Autodesk Fusion 360 part; units mm, degrees
(part 2 of 2)
sketch "oled" plane through (0, 0, 8) normal (0, 0, 1) x (-1, 0, 0)
  line L0 (-139.875, 29.334375) -> (-144.098992, 29.334375)
  line L1 (-144.644364, 25.834375) -> (-139.875, 25.834375)
  line L2 (-139.875, 25.834375) -> (-139.875, 23.834375)
  line L3 (-139.875, 23.834375) -> (-144.91061, 23.834375)
  line L4 (-145.297865, 20.334375) -> (-139.875, 20.334375)
  line L5 (-139.875, 20.334375) -> (-139.875, 18.334375)
  line L6 (-139.875, 18.334375) -> (-145.474496, 18.334375)
  line L7 (-145.705944, 14.834375) -> (-139.875, 14.834375)
  line L8 (-139.875, 14.834375) -> (-139.875, 12.834375)
  line L9 (-139.875, 12.834375) -> (-145.794002, 12.834375)
  line L10 (-145.871001, 9.334375) -> (-139.875, 9.334375)
  line L11 (-139.875, 9.334375) -> (-139.875, 7.334375)
  line L12 (-139.875, 7.334375) -> (-145.871001, 7.334375)
  line L13 (-145.794002, 3.834375) -> (-139.875, 3.834375)
  line L14 (-139.875, 3.834375) -> (-139.875, 1.834375)
  line L15 (-139.875, 1.834375) -> (-145.705944, 1.834375)
  line L16 (-145.474496, -1.665625) -> (-139.875, -1.665625)
  line L17 (-139.875, -1.665625) -> (-139.875, -3.665625)
  line L18 (-139.875, -3.665625) -> (-145.297865, -3.665625)
  line L19 (-144.91061, -7.165625) -> (-139.875, -7.165625)
  line L20 (-139.875, -7.165625) -> (-139.875, -9.165625)
  line L21 (-139.875, -9.165625) -> (-144.644364, -9.165625)
  line L22 (-144.098992, -12.665625) -> (-139.875, -12.665625)
  line L23 (-139.875, -12.665625) -> (-139.875, -14.665625)
  line L24 (-139.875, -14.665625) -> (-143.741524, -14.665625)
  line L25 (-143.034704, -18.165625) -> (-139.875, -18.165625)
  line L26 (-139.875, -18.165625) -> (-139.875, -20.165625)
  line L27 (-139.875, -20.165625) -> (-142.583799, -20.165625)
  line L28 (9.233799, -20.165625) -> (6.525, -20.165625)
  line L29 (6.525, -20.165625) -> (6.525, -18.165625)
  line L30 (6.525, -18.165625) -> (9.684704, -18.165625)
  line L31 (10.391524, -14.665625) -> (6.525, -14.665625)
  line L32 (6.525, -14.665625) -> (6.525, -12.665625)
  line L33 (6.525, -12.665625) -> (10.748992, -12.665625)
  line L34 (11.294364, -9.165625) -> (6.525, -9.165625)
  line L35 (6.525, -9.165625) -> (6.525, -7.165625)
  line L36 (6.525, -7.165625) -> (11.56061, -7.165625)
  line L37 (11.947865, -3.665625) -> (6.525, -3.665625)
  line L38 (6.525, -3.665625) -> (6.525, -1.665625)
  line L39 (6.525, -1.665625) -> (12.124496, -1.665625)
  line L40 (12.355944, 1.834375) -> (6.525, 1.834375)
  line L41 (6.525, 1.834375) -> (6.525, 3.834375)
  line L42 (6.525, 3.834375) -> (12.444002, 3.834375)
  line L43 (12.521001, 7.334375) -> (6.525, 7.334375)
  line L44 (6.525, 7.334375) -> (6.525, 9.334375)
  line L45 (6.525, 9.334375) -> (12.521001, 9.334375)
  line L46 (12.444002, 12.834375) -> (6.525, 12.834375)
  line L47 (6.525, 12.834375) -> (6.525, 14.834375)
  line L48 (6.525, 14.834375) -> (12.355944, 14.834375)
  line L49 (12.124496, 18.334375) -> (6.525, 18.334375)
  line L50 (6.525, 18.334375) -> (6.525, 20.334375)
  line L51 (6.525, 20.334375) -> (11.947865, 20.334375)
  line L52 (11.56061, 23.834375) -> (6.525, 23.834375)
  line L53 (6.525, 23.834375) -> (6.525, 25.834375)
  line L54 (6.525, 25.834375) -> (11.294364, 25.834375)
  line L55 (10.748992, 29.334375) -> (6.525, 29.334375)
  line L56 (6.525, 29.334375) -> (6.525, 31.334375)
  line L57 (6.525, 31.334375) -> (10.391524, 31.334375)
  line L58 (9.684704, 34.834375) -> (6.525, 34.834375)
  line L59 (6.525, 34.834375) -> (6.525, 36.834375)
  line L60 (6.525, 36.834375) -> (9.233799, 36.834375)
  line L61 (0.525, 41.625) -> (0.525, 19.525)
  arc A0 (-0.475, 18.525) -> (0.525, 19.525) centre (-0.475, 19.525) ccw
  line L62 (-0.475, 18.525) -> (-9, 18.525)
  line L63 (-9, 18.525) -> (-9, 0.475)
  arc A1 (-10, -0.525) -> (-9, 0.475) centre (-10, 0.475) ccw
  line L64 (-10, -0.525) -> (-47.15, -0.525)
  arc A2 (-48.15, 0.475) -> (-47.15, -0.525) centre (-47.15, 0.475) ccw
  line L65 (-48.15, 0.475) -> (-48.15, 18.525)
  line L66 (-48.15, 18.525) -> (-66.15, 18.525)
  line L67 (-66.15, 18.525) -> (-66.15, 0.475)
  arc A3 (-67.15, -0.525) -> (-66.15, 0.475) centre (-67.15, 0.475) ccw
  line L68 (-67.15, -0.525) -> (-123.35, -0.525)
  arc A4 (-124.35, 0.475) -> (-123.35, -0.525) centre (-123.35, 0.475) ccw
  line L69 (-124.35, 0.475) -> (-124.35, 18.525)
  line L70 (-124.35, 18.525) -> (-132.875, 18.525)
  arc A5 (-133.875, 19.525) -> (-132.875, 18.525) centre (-132.875, 19.525) ccw
  line L71 (-133.875, 19.525) -> (-133.875, 41.625)
  line L72 (-142.583799, 36.834375) -> (-139.875, 36.834375)
  line L73 (-139.875, 36.834375) -> (-139.875, 34.834375)
  line L74 (-139.875, 34.834375) -> (-143.034704, 34.834375)
  line L75 (-143.741524, 31.334375) -> (-139.875, 31.334375)
  line L76 (-139.875, 31.334375) -> (-139.875, 29.334375)
  circle A6 centre (-123.825, -13.096875) radius 10
  line L77 (-15.876065, -17.914896) -> (-3.386093, -17.890586)
  arc A7 (-3.381227, -20.390581) -> (-3.386093, -17.890586) centre (-3.38366, -19.140584) ccw
  line L78 (-3.381227, -20.390581) -> (-15.871199, -20.414891)
  arc A8 (-15.876065, -17.914896) -> (-15.871199, -20.414891) centre (-15.873632, -19.164893) ccw
  line L79 (-15.877503, -5.914899) -> (-3.387616, -5.876226)
  arc A9 (-3.379875, -8.376214) -> (-3.387616, -5.876226) centre (-3.383745, -7.12622) ccw
  line L80 (-3.379875, -8.376214) -> (-15.869762, -8.414887)
  arc A10 (-15.877503, -5.914899) -> (-15.869762, -8.414887) centre (-15.873632, -7.164893) ccw
  line L81 (-18.024549, -13.914894) -> (-1.172265, -13.895698)
  arc A11 (-1.169417, -16.395696) -> (-1.172265, -13.895698) centre (-1.170841, -15.145697) ccw
  line L82 (-1.169417, -16.395696) -> (-18.021701, -16.414893)
  arc A12 (-18.024549, -13.914894) -> (-18.021701, -16.414893) centre (-18.023125, -15.164893) ccw
  line L83 (-18.024544, -9.914894) -> (-1.172264, -9.895769)
  arc A13 (-1.169426, -12.395767) -> (-1.172264, -9.895768) centre (-1.170845, -11.145768) ccw
  line L84 (-1.169426, -12.395767) -> (-18.021707, -12.414893)
  arc A14 (-18.024544, -9.914894) -> (-18.021707, -12.414893) centre (-18.023125, -11.164893) ccw
  line L85 (-106.15, -6.096875) -> (-75.15, -6.096875)
  line L86 (-75.15, -20.096875) -> (-75.15, -6.096875)
  line L87 (-106.15, -20.096875) -> (-75.15, -20.096875)
  line L88 (-106.15, -20.096875) -> (-106.15, -6.096875)
  line L89 (-111.15, -5.096875) -> (-70.15, -5.096875)
  line L90 (-70.15, -21.096875) -> (-70.15, -5.096875)
  line L91 (-111.15, -21.096875) -> (-70.15, -21.096875)
  line L92 (-111.15, -21.096875) -> (-111.15, -5.096875)
  arc A15 (-144.098992, 29.334375) -> (-144.644364, 25.834375) centre (-20.832179, 8.334375) ccw
  arc A16 (-144.91061, 23.834375) -> (-145.297865, 20.334375) centre (-20.832179, 8.334375) ccw
  arc A17 (-145.474496, 18.334375) -> (-145.705944, 14.834375) centre (-20.832179, 8.334375) ccw
  arc A18 (-145.794002, 12.834375) -> (-145.871001, 9.334375) centre (-20.832179, 8.334375) ccw
  arc A19 (-145.871001, 7.334375) -> (-145.794002, 3.834375) centre (-20.832179, 8.334375) ccw
  arc A20 (-145.705944, 1.834375) -> (-145.474496, -1.665625) centre (-20.832179, 8.334375) ccw
  arc A21 (-145.297865, -3.665625) -> (-144.91061, -7.165625) centre (-20.832179, 8.334375) ccw
  arc A22 (-144.644364, -9.165625) -> (-144.098992, -12.665625) centre (-20.832179, 8.334375) ccw
  arc A23 (-143.741524, -14.665625) -> (-143.034704, -18.165625) centre (-20.832179, 8.334375) ccw
  arc A24 (-142.583799, -20.165625) -> (-141.563878, -24.216568) centre (-20.832179, 8.334375) ccw
  arc A25 (-141.563878, -24.216568) -> (-140.598355, -24.95625) centre (-140.598355, -23.95625) ccw
  line L93 (-140.598355, -24.95625) -> (7.248355, -24.95625)
  arc A26 (7.248355, -24.95625) -> (8.213878, -24.216568) centre (7.248355, -23.95625) ccw
  arc A27 (8.213878, -24.216568) -> (9.233799, -20.165625) centre (-112.517821, 8.334375) ccw
  arc A28 (9.684704, -18.165625) -> (10.391524, -14.665625) centre (-112.517821, 8.334375) ccw
  arc A29 (10.748992, -12.665625) -> (11.294364, -9.165625) centre (-112.517821, 8.334375) ccw
  arc A30 (11.56061, -7.165625) -> (11.947865, -3.665625) centre (-112.517821, 8.334375) ccw
  arc A31 (12.124496, -1.665625) -> (12.355944, 1.834375) centre (-112.517821, 8.334375) ccw
  arc A32 (12.444002, 3.834375) -> (12.521001, 7.334375) centre (-112.517821, 8.334375) ccw
  arc A33 (12.521001, 9.334375) -> (12.444002, 12.834375) centre (-112.517821, 8.334375) ccw
  arc A34 (12.355944, 14.834375) -> (12.124496, 18.334375) centre (-112.517821, 8.334375) ccw
  arc A35 (11.947865, 20.334375) -> (11.56061, 23.834375) centre (-112.517821, 8.334375) ccw
  arc A36 (11.294364, 25.834375) -> (10.748992, 29.334375) centre (-112.517821, 8.334375) ccw
  arc A37 (10.391524, 31.334375) -> (9.684704, 34.834375) centre (-112.517821, 8.334375) ccw
  arc A38 (9.233799, 36.834375) -> (8.213878, 40.885318) centre (-112.517821, 8.334375) ccw
  arc A39 (8.213878, 40.885318) -> (7.248355, 41.625) centre (7.248355, 40.625) ccw
  line L94 (7.248355, 41.625) -> (0.525, 41.625)
  line L95 (-133.875, 41.625) -> (-140.598355, 41.625)
  arc A40 (-140.598355, 41.625) -> (-141.563878, 40.885318) centre (-140.598355, 40.625) ccw
  arc A41 (-141.563878, 40.885318) -> (-142.583799, 36.834375) centre (-20.832179, 8.334375) ccw
  arc A42 (-143.034704, 34.834375) -> (-143.741524, 31.334375) centre (-20.832179, 8.334375) ccw
extrude "Extrude16" cut sketch "oled" against normal up to surface (4 mm away) contours L85 L86 L87 L88 picked at (-85.483333, -15.430208) bodies 2
extrude "Extrude17" cut sketch "oled" against normal up to surface (3.5 mm away) from surface at -0.5 contours L89 L90 L91 L92 picked at (-109.483333, -15.430208) bodies 2
chamfer "Chamfer1" distance 1 angle 45 16 edges at (9.624818, 8.39555, 4) (2.133751, 7.122349, 4) (9.632559, 5.895563, 4) (17.123626, 7.168764, 4) (9.598404, 9.905331, 4) (19.273124, 11.166312, 4) (9.595566, 12.40533, 4) (-0.079154, 11.144349, 4) (9.598407, 13.905296, 4) (19.273124, 15.166317, 4) (9.595559, 16.405294, 4) (-0.079158, 15.144273, 4) (9.631079, 17.902741, 4) (17.12363, 19.167326, 4) (9.626213, 20.402736, 4) (2.133662, 19.138151, 4) on bodies 2
extrude "Extrude18" cut sketch "top" along normal blind 6 contours A0 | A1 | A2 | A3 picked at (138.047024, 22.954852) picked at (-5.685457, -38.762887) picked at (138.48626, -39.612464) picked at (-5.495036, 21.990072) bodies 2
extrude "Extrude19" cut sketch "plate" against normal up to surface (3 mm away) contours A2 | A4 | A5 | A7 picked at (138.452882, 23.273596) picked at (-4.735816, -39.322162) picked at (-4.939523, 22.339037) picked at (138.297118, -39.942346) bodies 1
fillet "Fillet5" radius 1 8 edges at (-0.525, 21.95625, -1.5) (-0.525, 3.525, -1.5) (133.875, 21.95625, -1.5) (133.875, 3.525, -1.5) (66.65, 3.525, -1.5) (47.65, 3.525, -1.5) (47.65, -13.525, -1.5) (66.65, -13.525, -1.5) on bodies 1
fillet "Fillet6" radius 0.5 48 edges at (11.975, -2.45, -1.5) (26.125, -2.45, -1.5) (26.125, -16.6, -1.5) (11.975, -16.6, -1.5) (31.025, -16.6, -1.5) (31.025, -2.45, -1.5) (45.175, -2.45, -1.5) (45.175, -16.6, -1.5) (69.125, -2.45, -1.5) (83.275, -2.45, -1.5) (83.275, -16.6, -1.5) (69.125, -16.6, -1.5) (88.175, -2.45, -1.5) (102.325, -2.45, -1.5) (88.175, -16.6, -1.5) (102.325, -16.6, -1.5) (107.225, -2.45, -1.5) (121.375, -2.45, -1.5) (121.375, -16.6, -1.5) (107.225, -16.6, -1.5) (116.75, -21.5, -1.5) (130.9, -21.5, -1.5) (130.9, -35.65, -1.5) (116.75, -35.65, -1.5) (111.85, -35.772243, -1.5) (111.85, -21.5, -1.5) (97.7, -21.5, -1.5) (97.7, -35.772243, -1.5) (92.8, -35.65, -1.5) (92.8, -21.5, -1.5) (78.65, -21.5, -1.5) (78.65, -35.65, -1.5) (73.75, -35.65, -1.5) (73.75, -21.5, -1.5) (59.6, -21.5, -1.5) (59.6, -35.65, -1.5) (40.55, -21.5, -1.5) (54.7, -21.5, -1.5) (54.7, -35.65, -1.5) (40.55, -35.65, -1.5) (21.5, -21.5, -1.5) (35.65, -21.5, -1.5) (35.65, -35.65, -1.5) (21.5, -35.65, -1.5) (16.6, -35.65, -1.5) (16.6, -21.5, -1.5) (2.45, -21.5, -1.5) (2.45, -35.65, -1.5) on bodies 1
sketch "switchclip" plane through (0, 0, 0) normal (0, 0, 1) x (1, 0, 0)
  arc A0 (26.125, -2.45) -> (11.975, -2.45) centre (19.05, -18.385208) ccw
  arc A1 (11.975, -16.6) -> (26.125, -16.6) centre (19.05, -0.664792) ccw
  line L0 (11.975, -2.45) -> (11.975, -16.6)
  line L1 (26.125, -16.6) -> (26.125, -2.45)
  arc A2 (31.025, -16.6) -> (45.175, -16.6) centre (38.1, -0.664792) ccw
  line L2 (45.175, -16.6) -> (45.175, -2.45)
  arc A3 (45.175, -2.45) -> (31.025, -2.45) centre (38.1, -18.385208) ccw
  line L3 (31.025, -2.45) -> (31.025, -16.6)
  arc A4 (69.125, -16.6) -> (83.275, -16.6) centre (76.2, -0.664792) ccw
  line L4 (83.275, -16.6) -> (83.275, -2.45)
  arc A5 (83.275, -2.45) -> (69.125, -2.45) centre (76.2, -18.385208) ccw
  line L5 (69.125, -2.45) -> (69.125, -16.6)
  arc A6 (88.175, -16.6) -> (102.325, -16.6) centre (95.25, -0.664792) ccw
  line L6 (102.325, -16.6) -> (102.325, -2.45)
  arc A7 (102.325, -2.45) -> (88.175, -2.45) centre (95.25, -18.385208) ccw
  line L7 (88.175, -2.45) -> (88.175, -16.6)
  arc A8 (107.225, -16.6) -> (121.375, -16.6) centre (114.3, -0.664792) ccw
  line L8 (121.375, -16.6) -> (121.375, -2.45)
  arc A9 (121.375, -2.45) -> (107.225, -2.45) centre (114.3, -18.385208) ccw
  line L9 (107.225, -2.45) -> (107.225, -16.6)
  arc A10 (40.55, -35.65) -> (54.7, -35.65) centre (47.625, -19.714792) ccw
  arc A11 (54.7, -21.5) -> (40.55, -21.5) centre (47.625, -37.435208) ccw
  arc A12 (92.8, -21.5) -> (78.65, -21.5) centre (85.725, -37.435208) ccw
  line L10 (35.65, -35.65) -> (35.65, -21.5)
  arc A13 (116.75, -35.65) -> (130.9, -35.65) centre (123.825, -19.714792) ccw
  line L11 (40.55, -21.5) -> (40.55, -35.65)
  line L12 (21.5, -21.5) -> (21.5, -35.65)
  arc A14 (97.7, -35.65) -> (111.85, -35.65) centre (104.775, -19.714792) ccw
  arc A15 (78.65, -35.65) -> (92.8, -35.65) centre (85.725, -19.714792) ccw
  line L13 (78.65, -21.5) -> (78.65, -35.65)
  arc A16 (35.65, -21.5) -> (21.5, -21.5) centre (28.575, -37.435208) ccw
  arc A17 (16.6, -21.5) -> (2.45, -21.5) centre (9.525, -37.435208) ccw
  line L14 (59.6, -21.5) -> (59.6, -35.65)
  line L15 (54.7, -35.65) -> (54.7, -21.5)
  line L16 (130.9, -35.65) -> (130.9, -21.5)
  arc A18 (59.6, -35.65) -> (73.75, -35.65) centre (66.675, -19.714792) ccw
  arc A19 (2.45, -35.65) -> (16.6, -35.65) centre (9.525, -19.714792) ccw
  arc A20 (73.75, -21.5) -> (59.6, -21.5) centre (66.675, -37.435208) ccw
  line L17 (97.7, -21.5) -> (97.7, -35.65)
  line L18 (2.45, -21.5) -> (2.45, -35.65)
  arc A21 (21.5, -35.65) -> (35.65, -35.65) centre (28.575, -19.714792) ccw
  line L19 (111.85, -35.65) -> (111.85, -21.5)
  line L20 (92.8, -35.65) -> (92.8, -21.5)
  line L21 (16.6, -35.65) -> (16.6, -21.5)
  line L22 (73.75, -35.65) -> (73.75, -21.5)
  arc A22 (130.9, -21.5) -> (116.75, -21.5) centre (123.825, -37.435208) ccw
  arc A23 (111.85, -21.5) -> (97.7, -21.5) centre (104.775, -37.435208) ccw
  line L23 (116.75, -21.5) -> (116.75, -35.65)
  dimension "d151" = 19.05
  dimension "d152" = 0
  dimension "d155" = 19.05
  dimension "d156" = 0
  constraint vertical L0
  constraint parallel L0 L1
  constraint vertical L18
  constraint parallel L18 L21
extrude "Extrude20" cut sketch "switchclip" against normal up to surface (1.5 mm away) from surface at -1.5 contours A0 A1 L0 L1 | A2 L2 A3 L3 | A4 L4 A5 L5 | A6 L6 A7 L7 | A8 L8 A9 L9 | A10 A11 L11 L15 | A12 A15 L13 L20 | L10 L12 A16 A21 | A13 L16 A22 L23 | A14 L17 L19 A23 | A17 A19 L18 L21 | L14 A18 A20 L22 picked at (18.243154, -12.327053) picked at (38.906846, -12.327053) picked at (75.393154, -12.327053) picked at (94.443154, -12.327053) picked at (113.493154, -12.327053) picked at (46.818154, -31.377053) picked at (84.918154, -31.377053) picked at (29.381846, -31.377053) picked at (123.018154, -25.772947) picked at (103.968154, -25.772947) picked at (10.331846, -25.772947) picked at (65.868154, -25.772947) bodies 1
extrude "Extrude21" cut sketch "bottom" against normal up to surface (11 mm away) contours A6 | A7 | A8 | A9 picked at (-4.939523, 22.339037) picked at (138.452882, 21.638904) picked at (138.297118, -38.307654) picked at (-4.735816, -39.322162) bodies 3
extrude "Extrude22" cut sketch "bottom" against normal up to surface (5 mm away) from surface at -6 contours A0 | A1 | A2 | A3 picked at (137.757246, 20.542276) picked at (-3.02155, 22.279883) picked at (-3.017641, -39.249202) picked at (137.757246, -41.038974) bodies 3
sketch "bumpons" plane through (0, 0, -11) normal (0, 0, -1) x (1, 0, 0)
  circle A0 centre (-5.025, 39.125) radius 2.5
  circle A1 centre (138.375, 39.125) radius 2.5
  circle A2 centre (-5.025, -22.45625) radius 2.5
  circle A3 centre (138.375, -22.45625) radius 2.5
  line L0 (139.875, 25.834375) -> (144.644364, 25.834375)
  line L1 (144.098992, 29.334375) -> (139.875, 29.334375)
  line L2 (139.875, 29.334375) -> (139.875, 31.334375)
  line L3 (139.875, 31.334375) -> (143.741524, 31.334375)
  line L4 (143.034704, 34.834375) -> (139.875, 34.834375)
  line L5 (139.875, 34.834375) -> (139.875, 36.834375)
  line L6 (139.875, 36.834375) -> (142.583799, 36.834375)
  line L7 (-9.233799, 36.834375) -> (-6.525, 36.834375)
  line L8 (-6.525, 36.834375) -> (-6.525, 34.834375)
  line L9 (-6.525, 34.834375) -> (-9.684704, 34.834375)
  line L10 (-10.391524, 31.334375) -> (-6.525, 31.334375)
  line L11 (-6.525, 31.334375) -> (-6.525, 29.334375)
  line L12 (-6.525, 29.334375) -> (-10.748992, 29.334375)
  line L13 (-11.294364, 25.834375) -> (-6.525, 25.834375)
  line L14 (-6.525, 25.834375) -> (-6.525, 23.834375)
  line L15 (-6.525, 23.834375) -> (-11.56061, 23.834375)
  line L16 (-11.947865, 20.334375) -> (-6.525, 20.334375)
  line L17 (-6.525, 20.334375) -> (-6.525, 18.334375)
  line L18 (-6.525, 18.334375) -> (-12.124496, 18.334375)
  line L19 (-12.355944, 14.834375) -> (-6.525, 14.834375)
  line L20 (-6.525, 14.834375) -> (-6.525, 12.834375)
  line L21 (-6.525, 12.834375) -> (-12.444002, 12.834375)
  line L22 (-12.521001, 9.334375) -> (-6.525, 9.334375)
  line L23 (-6.525, 9.334375) -> (-6.525, 7.334375)
  line L24 (-6.525, 7.334375) -> (-12.521001, 7.334375)
  line L25 (-12.444002, 3.834375) -> (-6.525, 3.834375)
  line L26 (-6.525, 3.834375) -> (-6.525, 1.834375)
  line L27 (-6.525, 1.834375) -> (-12.355944, 1.834375)
  line L28 (-12.124496, -1.665625) -> (-6.525, -1.665625)
  line L29 (-6.525, -1.665625) -> (-6.525, -3.665625)
  line L30 (-6.525, -3.665625) -> (-11.947865, -3.665625)
  line L31 (-11.56061, -7.165625) -> (-6.525, -7.165625)
  line L32 (-6.525, -7.165625) -> (-6.525, -9.165625)
  line L33 (-6.525, -9.165625) -> (-11.294364, -9.165625)
  line L34 (-10.748992, -12.665625) -> (-6.525, -12.665625)
  line L35 (-6.525, -12.665625) -> (-6.525, -14.665625)
  line L36 (-6.525, -14.665625) -> (-10.391524, -14.665625)
  line L37 (-9.684704, -18.165625) -> (-6.525, -18.165625)
  line L38 (-6.525, -18.165625) -> (-6.525, -20.165625)
  line L39 (-6.525, -20.165625) -> (-9.233799, -20.165625)
  line L40 (142.583799, -20.165625) -> (139.875, -20.165625)
  line L41 (139.875, -20.165625) -> (139.875, -18.165625)
  line L42 (139.875, -18.165625) -> (143.034704, -18.165625)
  line L43 (143.741524, -14.665625) -> (139.875, -14.665625)
  line L44 (139.875, -14.665625) -> (139.875, -12.665625)
  line L45 (139.875, -12.665625) -> (144.098992, -12.665625)
  line L46 (144.644364, -9.165625) -> (139.875, -9.165625)
  line L47 (139.875, -9.165625) -> (139.875, -7.165625)
  line L48 (139.875, -7.165625) -> (144.91061, -7.165625)
  line L49 (145.297865, -3.665625) -> (139.875, -3.665625)
  line L50 (139.875, -3.665625) -> (139.875, -1.665625)
  line L51 (139.875, -1.665625) -> (145.474496, -1.665625)
  line L52 (145.705944, 1.834375) -> (139.875, 1.834375)
  line L53 (139.875, 1.834375) -> (139.875, 3.834375)
  line L54 (139.875, 3.834375) -> (145.794002, 3.834375)
  line L55 (145.871001, 7.334375) -> (139.875, 7.334375)
  line L56 (139.875, 7.334375) -> (139.875, 9.334375)
  line L57 (139.875, 9.334375) -> (145.871001, 9.334375)
  line L58 (145.794002, 12.834375) -> (139.875, 12.834375)
  line L59 (139.875, 12.834375) -> (139.875, 14.834375)
  line L60 (139.875, 14.834375) -> (145.705944, 14.834375)
  line L61 (145.474496, 18.334375) -> (139.875, 18.334375)
  line L62 (139.875, 18.334375) -> (139.875, 20.334375)
  line L63 (139.875, 20.334375) -> (145.297865, 20.334375)
  line L64 (144.91061, 23.834375) -> (139.875, 23.834375)
  line L65 (139.875, 23.834375) -> (139.875, 25.834375)
  circle A4 centre (3.046068, -19.95625) radius 4.5
  circle A5 centre (3.046068, 36.625) radius 4.5
  circle A6 centre (130.303932, 36.625) radius 4.5
  circle A7 centre (130.303932, -19.95625) radius 4.5
  arc A8 (144.644364, 25.834375) -> (144.098992, 29.334375) centre (20.832179, 8.334375) ccw
  arc A9 (143.741524, 31.334375) -> (143.034704, 34.834375) centre (20.832179, 8.334375) ccw
  arc A10 (142.583799, 36.834375) -> (141.563878, 40.885318) centre (20.832179, 8.334375) ccw
  arc A11 (141.563878, 40.885318) -> (140.598355, 41.625) centre (140.598355, 40.625) ccw
  line L66 (140.598355, 41.625) -> (138.375, 41.625)
  line L67 (138.375, 41.625) -> (-5.025, 41.625)
  line L68 (-5.025, 41.625) -> (-7.248355, 41.625)
  arc A12 (-7.248355, 41.625) -> (-8.213878, 40.885318) centre (-7.248355, 40.625) ccw
  arc A13 (-8.213878, 40.885318) -> (-9.233799, 36.834375) centre (112.517821, 8.334375) ccw
  arc A14 (-9.684704, 34.834375) -> (-10.391524, 31.334375) centre (112.517821, 8.334375) ccw
  arc A15 (-10.748992, 29.334375) -> (-11.294364, 25.834375) centre (112.517821, 8.334375) ccw
  arc A16 (-11.56061, 23.834375) -> (-11.947865, 20.334375) centre (112.517821, 8.334375) ccw
  arc A17 (-12.124496, 18.334375) -> (-12.355944, 14.834375) centre (112.517821, 8.334375) ccw
  arc A18 (-12.444002, 12.834375) -> (-12.521001, 9.334375) centre (112.517821, 8.334375) ccw
  arc A19 (-12.521001, 7.334375) -> (-12.444002, 3.834375) centre (112.517821, 8.334375) ccw
  arc A20 (-12.355944, 1.834375) -> (-12.124496, -1.665625) centre (112.517821, 8.334375) ccw
  arc A21 (-11.947865, -3.665625) -> (-11.56061, -7.165625) centre (112.517821, 8.334375) ccw
  arc A22 (-11.294364, -9.165625) -> (-10.748992, -12.665625) centre (112.517821, 8.334375) ccw
  arc A23 (-10.391524, -14.665625) -> (-9.684704, -18.165625) centre (112.517821, 8.334375) ccw
  arc A24 (-9.233799, -20.165625) -> (-8.213878, -24.216568) centre (112.517821, 8.334375) ccw
  arc A25 (-8.213878, -24.216568) -> (-7.248355, -24.95625) centre (-7.248355, -23.95625) ccw
  line L69 (-7.248355, -24.95625) -> (-5.025, -24.95625)
  line L70 (-5.025, -24.95625) -> (138.375, -24.95625)
  line L71 (138.375, -24.95625) -> (140.598355, -24.95625)
  arc A26 (140.598355, -24.95625) -> (141.563878, -24.216568) centre (140.598355, -23.95625) ccw
  arc A27 (141.563878, -24.216568) -> (142.583799, -20.165625) centre (20.832179, 8.334375) ccw
  arc A28 (143.034704, -18.165625) -> (143.741524, -14.665625) centre (20.832179, 8.334375) ccw
  arc A29 (144.098992, -12.665625) -> (144.644364, -9.165625) centre (20.832179, 8.334375) ccw
  arc A30 (144.91061, -7.165625) -> (145.297865, -3.665625) centre (20.832179, 8.334375) ccw
  arc A31 (145.474496, -1.665625) -> (145.705944, 1.834375) centre (20.832179, 8.334375) ccw
  arc A32 (145.794002, 3.834375) -> (145.871001, 7.334375) centre (20.832179, 8.334375) ccw
  arc A33 (145.871001, 9.334375) -> (145.794002, 12.834375) centre (20.832179, 8.334375) ccw
  arc A34 (145.705944, 14.834375) -> (145.474496, 18.334375) centre (20.832179, 8.334375) ccw
  arc A35 (145.297865, 20.334375) -> (144.91061, 23.834375) centre (20.832179, 8.334375) ccw
  dimension "d207" = 9
  measures "d207" diameter of A4
extrude "Extrude23" cut sketch "bumpons" against normal blind 0.5 contours A4 | A5 | A6 | A7 picked at (4.916537, -22.301744) picked at (2.110833, 38.244874) picked at (131.597511, 38.932372) picked at (131.597511, -17.648878) bodies 3
fillet "Fillet7" radius 1 4 edges at (-0.525, 21.95625, 2) (-0.525, 3.525, 2) (133.875, 3.525, 2) (133.875, 21.95625, 2) on bodies 2
fillet "Fillet8" radius 1 4 edges at (106.15, 20.096875, 7.75) (106.15, 6.096875, 7.75) (75.15, 6.096875, 7.75) (75.15, 20.096875, 7.75) on bodies 2
fillet "Fillet9" radius 0.5 4 edges at (48.15, -18.525, 4) (9, -18.525, 4) (66.15, -18.525, 4) (124.35, -18.525, 4) on bodies 2
extrude "Extrude24" cut sketch "plate" along normal blind 9 from surface at -6 contours L70 L71 L74 L75 A8 A9 A10 A11 | L72 L73 L76 L77 A12 A13 A14 A15 picked at (44.483333, 24.122917) picked at (69.816667, 24.122917) bodies 1 2 3
extrude "Extrude25" add sketch "plate" along normal blind 1.8 separate body contours L78 L79 L80 L81 picked at (162.666669, 2) makes body 4
extrude "Extrude26" cut sketch "usb" against normal up to surface (1.5 mm away) from surface at -40.48125 contours L8 L9 L10 L11 picked at (55.9, -3.833333) bodies 3
equation "depth = 1 mm"
named bodies: "pianissimo_plate", "pianissimo_top", "pianissimo_bottom", "pianissimo_peg"
